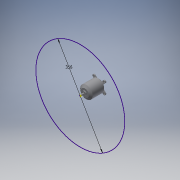
# Autodesk Inventor part: Motor Turnigy G60 500kv
Saved by Autodesk Inventor 2018 (Build 220112000, 112)
## iProperties
Created: 2018-07-21
Part Number: Motor Turnigy G60 500kv
Material: Generic
Document SubType Name: Modeling
Designer: Michael Gunderman
Density: 3.67534 g/cm^3
Appearance: Default
Mass: 410 g
Surface Area: 140.751 cm^2
Volume: 111.554 cm^3
Author: Michael Gunderman
Autodesk Inventor part; units mm, degrees
ref_plane "YZ Plane" through (0, 0, 0) normal (1, 0, 0) x (0, 1, 0)
ref_plane "XZ Plane" through (0, 0, 0) normal (0, 1, 0) x (-1, 0, 0)
ref_plane "XY Plane" through (0, 0, 0) normal (0, 0, 1) x (1, 0, 0)
sketch "Sketch1" plane through (0, 0, 0) normal (0, 0, 1) x (1, 0, 0)
  line L0 (0, 0) -> (-20.7182, 20.7182) construction
  line L1 (7.0711, 0) -> (29.3, 0) construction
  line L2 (0, 0) -> (20.7182, 20.7182) construction
  line L3 (0, 0) -> (29.3, 0) construction
  line L4 (-20.7182, 20.7182) -> (20.7182, 20.7182) construction
  circle A0 centre (-20.7182, 20.7182) radius 2.5
  circle A1 centre (20.7182, 20.7182) radius 2.5
  circle A2 centre (-20.7182, -20.7182) radius 2.5
  circle A3 centre (20.7182, -20.7182) radius 2.5
  arc A4 (-24.2538, -17.1827) -> (-17.1827, -24.2538) centre (-20.7182, -20.7182) ccw
  line L5 (20.7182, 20.7182) -> (13.788, 27.6485) construction
  arc A5 (24.2538, 17.1827) -> (17.1827, 24.2538) centre (20.7182, 20.7182) ccw
  arc A6 (-17.1827, 24.2538) -> (-24.2538, 17.1827) centre (-20.7182, 20.7182) ccw
  arc A7 (17.1827, -24.2538) -> (24.2538, -17.1827) centre (20.7182, -20.7182) ccw
  line L6 (17.1827, 24.2538) -> (0, 7.0711)
  line L7 (-7.0711, 0) -> (-24.2538, -17.1827)
  line L8 (24.2538, -17.1827) -> (7.0711, 0)
  line L9 (0, 7.0711) -> (-17.1827, 24.2538)
  line L10 (24.2538, 17.1827) -> (7.0711, 0)
  line L11 (0, -7.0711) -> (-17.1827, -24.2538)
  line L12 (17.1827, -24.2538) -> (0, -7.0711)
  line L13 (-7.0711, 0) -> (-24.2538, 17.1827)
  dimension "d0" = 29.3
  dimension "d1" = 135
  dimension "d2" = 29.3
  dimension "d3" = 45
  dimension "d4" = 2.5
  dimension "d5" = 2.5
  dimension "d6" = 5
  dimension "d7" = 5
  constraints: 28 end point, 8 centre point, 8 point on circle, 7 symmetric about line, 4 coincident, 4 tangent, 2 horizontal, 2 point on line, 1 equal length, 1 perpendicular, 4 other
  measures "d0" distance of L0.start L0.end
  measures "d1" angle of L1 L0
  measures "d2" distance of L0.start L2.end
  measures "d3" angle of L3 L2
  measures "d4" radius of A0
  measures "d5" radius of A1
  measures "d6" radius of A4
  measures "d7" radius of A5
extrude "Extrusion1" add sketch "Sketch1" along normal blind 4
sketch "Sketch2" plane through (0, 0, 4) normal (0, 0, 1) x (1, 0, 0)
  circle A0 centre (0, 0) radius 25.01
  dimension "d10" = 25.01
  constraints: 1 centre point, 1 coincident
  measures "d10" radius of A0
extrude "Extrusion2" add sketch "Sketch2" along normal blind 50
chamfer "Chamfer1" distance 4 angle 45 5 edges at (23.9509, 7.201, 4) (23.9509, -7.201, 4) (0, -25.01, 4) (-25.01, 0, 4) (0, 25.01, 4)
sketch "Sketch3" plane through (0, 0, 54) normal (0, 0, 1) x (1, 0, 0)
  line L0 (0, 0) -> (25.01, 0)
  circle A0 centre (0, 0) radius 25.01 projected
  constraints: 2 end point, 1 horizontal, 1 horizontal alignment, 1 other
sketch "Sketch4" plane through (0, 0, 0) normal (0, 0, -1) x (-1, 0, 0)
  point P0 (0, 0)
  point P1 (0, 0)
  constraints: 1 coincident
ref_plane "Work Plane1" through (0, 0, 0) normal (0, 1, 0) x (0, 0, 1)
sketch "Sketch5" plane through (0, 0, 0) normal (0, 1, 0) x (0, 0, 1)
  line L0 (54, -25.01) -> (54, 25.01) projected
  line L1 (54, 0) -> (79, 0)
  line L2 (79, 0) -> (79, 3)
  line L3 (79, 3) -> (64, 3)
  line L4 (64, 3) -> (64, 8)
  line L5 (64, 8) -> (60.25, 8)
  line L6 (60.25, 8) -> (60.25, 16)
  line L7 (60.25, 16) -> (54, 25.01)
  point P0 (0, 0)
  dimension "d16" = 25
  dimension "d17" = 3
  dimension "d18" = 15
  dimension "d19" = 5
  dimension "d20" = 3.75
  dimension "d21" = 8
  constraints: 14 end point, 4 perpendicular, 1 horizontal, 1 midpoint, 1 vertical
  measures "d16" distance of L1.start L1.end
  measures "d17" distance of L1.end L2.end
  measures "d18" distance of L2.end L3.end
  measures "d19" distance of L3.end L4.end
  measures "d20" distance of L4.end L5.end
  measures "d21" distance of L5.end L6.end
revolve "Revolution1" add sketch "Sketch5" angle 360 about axis through (0, 0, 54) along (0, 0, 1)
sketch "Sketch6" plane through (0, 0, 79) normal (0, 0, 1) x (1, 0, 0)
  circle A0 centre (0, 0) radius 3 projected
  circle A1 centre (0, 0) radius 178
  dimension "d23" = 356
  constraints: 1 centre point, 1 coincident
  measures "d23" diameter of A1
body "Solid1"
